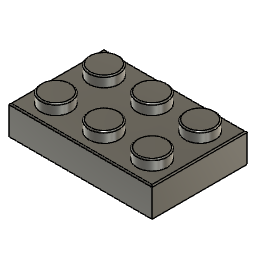
2x3block (Autodesk Fusion 360 design; units mm, degrees)
Autodesk Fusion 360 part; units mm, degrees
sketch "Sketch1" plane through (0, 0, 0) normal (0, 0, 1) x (1, 0, 0)
  line L0 (0, 0) -> (23.8, 0)
  line L1 (23.8, 0) -> (23.8, 15.8)
  line L2 (23.8, 15.8) -> (0, 15.8)
  line L3 (0, 15.8) -> (0, 0)
  constraint coincident L0.start L3.end
extrude "Extrude1" add sketch "Sketch1" along normal blind 4.8
sketch "Sketch2" plane through (0, 0, 4.8) normal (0, 0, 1) x (-1, 0, 0)
  line L0 (0, -15.8) -> (0, 0)
  line L1 (0, 0) -> (-23.8, 0)
  line L2 (-23.8, 0) -> (-23.8, -15.8)
  line L3 (-23.8, -15.8) -> (0, -15.8)
  circle A0 centre (-3.9, -11.9) radius 2.5
extrude "Extrude2" add sketch "Sketch2" along normal blind 1.7 contours A0
pattern_linear "R-Pattern1" count 3 spacing 8 along (1, 0, 0) count 2 spacing 8 along (0, -1, 0) of "Extrude2"
shell "Shell1" thickness 1.49 removed faces 1 at (7.9333, 10.5333, 0)
sketch "Sketch3" plane through (0, 0, 3.31) normal (0, 0, -1) x (1, 0, 0)
  circle A0 centre (19.9, -3.9) radius 1.01
  circle A1 centre (11.9, -3.9) radius 1.01
  circle A2 centre (3.9, -3.9) radius 1.01
  circle A3 centre (19.9, -11.9) radius 1.01
  circle A4 centre (11.9, -11.9) radius 1.01
  circle A5 centre (3.9, -11.9) radius 1.01
  line L0 (1.49, -1.49) -> (1.49, -14.31)
  line L1 (1.49, -14.31) -> (22.31, -14.31)
  line L2 (22.31, -14.31) -> (22.31, -1.49)
  line L3 (22.31, -1.49) -> (1.49, -1.49)
  circle A6 centre (7.9, -7.9) radius 3.15
  circle A7 centre (7.9, -7.9) radius 2.15
extrude "Extrude3" add sketch "Sketch3" along normal blind 3.3 contours A6
pattern_linear "R-Pattern2" count 2 spacing 8 along (1, 0, 0) of "Extrude3"
fillet "Fillet1" radius 0.2 10 edges at (0, 7.9, 4.8) (11.9, 15.8, 4.8) (11.9, 0, 4.8) (23.8, 7.9, 4.8) (22.2308, 4.804, 6.5) (22.2308, 12.804, 6.5) (14.2308, 12.804, 6.5) (14.2308, 4.804, 6.5) (6.2308, 4.804, 6.5) (6.2308, 12.804, 6.5)
scale "Scale1" factor 0.75 about (0.2, 15.6, 4.8) bodies 1
